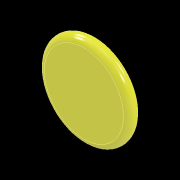
# Autodesk Inventor part: 模擬錢幣
Saved by Autodesk Inventor 2020 (Build 240168000, 168)
## iProperties
Created: 2021-04-13
Part Number: 模擬錢幣
Material: 一般
Document SubType Name: Modeling
Designer: 88690
Density: 1 g/cm^3
Appearance: 黃
Author: 88690
Autodesk Inventor part; units mm, degrees
ref_plane "XZ Plane" through (0, 0, 0) normal (0, 1, 0) x (-1, 0, 0)
ref_plane "XY Plane" through (0, 0, 0) normal (0, 0, 1) x (1, 0, 0)
sketch "草圖1" plane through (0, 0, 0) normal (0, 0, 1) x (1, 0, 0)
  circle A0 centre (0, 0) radius 15
  dimension "d0" = 30
  constraints: 1 centre point, 1 coincident
  measures "d0" diameter of A0
extrude "擠出1" add sketch "草圖1" along normal mid plane 4
fillet "圓角1" radius 2 2 edges at (-15, 0, 2) (-15, 0, -2)
ref_plane "工作平面1" through (15, 0, 0) normal (1, 0, 0) x (0, 1, 0)
